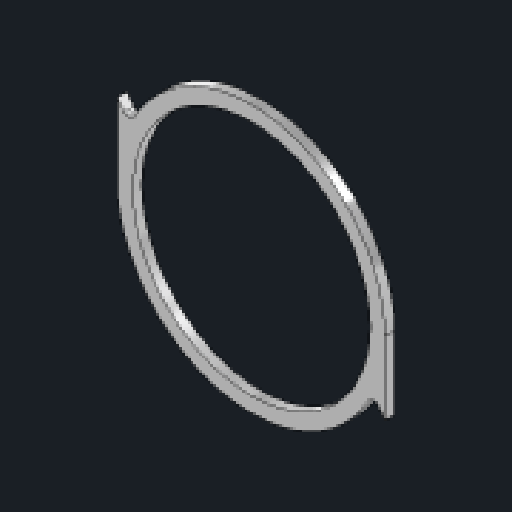
# Autodesk Inventor part: Weapon
Saved by Autodesk Inventor 2023.2 (Build 272271030, 271C)
## iProperties
Created: 2024-03-01
Part Number: Weapon
Material: Aluminum 6061
Document SubType Name: Modeling
Designer: robpl
Density: 2.7 g/cm^3
Appearance: Aluminum - Flat
Mass: 48.4899 g
Surface Area: 115.829 cm^2
Volume: 17.9592 cm^3
Author: robpl
Autodesk Inventor part; units mm, degrees
ref_plane "YZ Plane" through (0, 0, 0) normal (1, 0, 0) x (0, 1, 0)
ref_plane "XZ Plane" through (0, 0, 0) normal (0, 1, 0) x (-1, 0, 0)
ref_plane "XY Plane" through (0, 0, 0) normal (0, 0, 1) x (1, 0, 0)
sketch "Sketch1" plane through (0, 0, 0) normal (0, 0, 1) x (1, 0, 0)
  circle A0 centre (0, 0) radius 63.5
  circle A1 centre (0, 0) radius 71.5
  line L0 (-71.5, 0) -> (-71.5, 39.1152)
  line L1 (-71.5, 39.1152) -> (0, 0)
  line L2 (-71.5, 39.1152) -> (-65.0238, 29.7348)
  arc A2 (-67.9977, 34.0424) -> (-62.727, 34.3158) centre (-65.4466, 35.8036) ccw
  arc A3 (67.9977, -34.0424) -> (62.727, -34.3158) centre (65.4466, -35.8036) ccw
  line L3 (71.5, -39.1152) -> (65.0238, -29.7348)
  line L4 (71.5, 0) -> (71.5, -39.1152)
  point P0 (71.5, 0)
  dimension "d0" = 127
  dimension "d1" = 8
  dimension "d4" = 10
  dimension "d5" = 3.1
  dimension "d8" = 360
  constraints: 10 end point, 7 point on circle, 4 centre point, 3 point on line, 3 tangent, 1 coincident, 1 vertical, 19 other
  measures "d0" diameter of A0
  measures "d1" radial gap between concentric circles of A0 A1
  measures "d4" distance of L0.end A1.end
  measures "d5" radius of A2
extrude "Extrusion1" add sketch "Sketch1" along normal blind 5 contours A1 | L4 L3 A1 | A1 L2 A2 | L3 A3 A1 | A1 L0 L2
body "Solid1"
